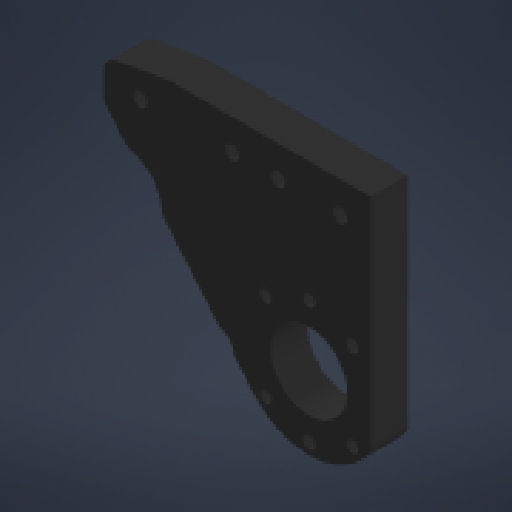
# Autodesk Inventor part: OUTSIDE_INTAKE_SPACERS
Saved by Autodesk Inventor 2026.2 (Build 302298010, 298A)
## iProperties
Created: 2026-04-02
Part Number: OUTSIDE_INTAKE_SPACERS
Material: 3D Print Material - chopped carbon Nylon12 (preferred)
Document SubType Name: Modeling
Designer: 4aida
Density: 1.05184 g/cm^3
Appearance: Black
Author: 4aida
Autodesk Inventor part; units mm, degrees
ref_plane "YZ Plane" through (0, 0, 0) normal (1, 0, 0) x (0, 1, 0)
ref_plane "XZ Plane" through (0, 0, 0) normal (0, 1, 0) x (-1, 0, 0)
ref_plane "XY Plane" through (0, 0, 0) normal (0, 0, 1) x (1, 0, 0)
sketch "Sketch1" plane through (0, 0, 0) normal (0, 0, 1) x (1, 0, 0)
  line L0 (-110, -20.8494) -> (-110, 0)
  line L1 (-110, 0) -> (0, 0)
  line L2 (0, 0) -> (0, -105)
  line L3 (0, -105) -> (-39.3892, -105)
  line L4 (-110, -20.8494) -> (-119.38, 0) construction
  line L5 (-119.38, 0) -> (-110, 0) construction
  line L6 (-50.8, -25.4) -> (0, -25.4) construction
  line L7 (0, -25.4) -> (0, 0) construction
  line L8 (0, 0) -> (-50.8, 0) construction
  line L9 (-50.8, 0) -> (-50.8, -25.4) construction
  line L10 (-50.8, -25.4) -> (0, 0) construction
  line L11 (0, -25.4) -> (-50.8, 0) construction
  circle A0 centre (-12.7, -12.7) radius 3
  circle A1 centre (-38.1, -12.7) radius 3
  circle A2 centre (-25.4, -75) radius 15.875
  circle A3 centre (-25.4, -75) radius 30
  line L12 (-50.8, -90.9637) -> (-50.8, -59.0363)
  line L13 (-110, -4.7091) -> (-83.2932, 0)
  arc A4 (-56.3982, -84.7295) -> (-61.7755, -78.3211) centre (-62.3821, -84.2903) ccw
  line L14 (-39.3892, -105) -> (-56.3982, -84.7295)
  arc A5 (-85.9963, -49.4559) -> (-100.0831, -32.6679) centre (-102.5, -49) ccw
  line L15 (-61.7755, -78.3211) -> (-85.9963, -49.4559)
  line L16 (-100.0831, -32.6679) -> (-110, -20.8494)
  circle A6 centre (-95.25, -12.7) radius 3
  circle A7 centre (-57.15, -12.7) radius 3
  point P0 (0, 0)
  point P1 (-25.4, -12.7)
  point P2 (-25.4, -25.4)
  point P3 (-50.8, -75)
  point P4 (0, -90.9637)
  point P5 (-110, -10.4247)
  point P6 (-48.3813, -94.2836)
  point P7 (0, -59.0363)
  point P8 (-25.4, -105)
  dimension "d1" = 119.38
  dimension "d2" = 50.8
  dimension "d3" = 25.4
  dimension "d4" = 25.4
  dimension "d5" = 12.7
  dimension "d6" = 6
  dimension "d7" = 6
  dimension "d11" = 110
  dimension "d12" = 60
  dimension "d13" = 25.4
  dimension "d14" = 25.4
  dimension "d17" = 20.8494
  dimension "d18" = 31.75
  dimension "d21" = 170
  dimension "d22" = 26.7068
  dimension "d24" = 86.6409
  dimension "d25" = 12
  dimension "d26" = 47.6179
  dimension "d28" = 81.3659
  dimension "d29" = 33.02
  dimension "d30" = 49
  dimension "d31" = 50
  dimension "d41" = 19.05
  dimension "d42" = 38.1
  constraints: 34 end point, 8 centre point, 6 point on circle, 5 midpoint, 4 horizontal alignment, 4 perpendicular, 4 tangent, 3 coincident, 2 collinear, 2 equal radius, 2 horizontal, 2 parallel, 2 point on line, 2 vertical, 1 vertical alignment
  measures "d1" distance from line of L2 L4.end
  measures "d2" distance of L6.start L6.end
  measures "d3" distance of L11.end L6.start
  measures "d4" distance of A1.centre A0.centre
  measures "d5" distance of point (-25.4, -12.7) A0.centre
  measures "d6" diameter of A0
  measures "d7" diameter of A1
  measures "d11" distance between parallel lines of L2 L0
  measures "d12" diameter of A3
  measures "d13" distance from line of A2.centre L2
  measures "d14" distance of point (-50.8, -75) A2.centre
  measures "d17" distance of L0.start L1.start
  measures "d18" diameter of A2
  measures "d21" angle of L13 L1
  measures "d22" horizontal distance of point (-110, -10.425) L13.end
  measures "d24" distance from line of L13 A4.centre
  measures "d25" diameter of A4
  measures "d26" distance from line of A4.centre L0
  measures "d28" distance of A5.centre A3.centre
  measures "d29" diameter of A5
  measures "d30" distance from line of L1 A5.centre
  measures "d31" angle of L1 L15
  measures "d41" distance of A1.centre A7.centre
  measures "d42" distance of A7.centre A6.centre
extrude "Extrusion1" add sketch "Sketch1" along normal blind 15.4305 contours L0 L13 L1 L2 A3 L14 A4 L15 A5 L16 | L2 A3 L12 | L12 A3
fillet "Fillet1" radius 6 8 edges at (0, -90.9637, 7.7153) (-110, -20.8494, 7.7153) (-110, -4.7091, 7.7153) (-83.2932, 0, 7.7153) (-56.3982, -84.7295, 7.7153) (-61.7755, -78.3211, 7.7153) (-85.9963, -49.4559, 7.7153) (-100.0831, -32.6679, 7.7153)
sketch "Sketch2" plane through (0, 0, 0) normal (0, 0, -1) x (-1, 0, 0)
  circle A0 centre (25.4, -75) radius 15.875 projected
  circle A1 centre (25.4, -75) radius 25.4
  line L0 (7.4395, -92.9605) -> (7.4395, -57.0395)
  line L1 (43.3605, -57.0395) -> (43.3605, -92.9605)
  line L2 (7.4395, -92.9605) -> (25.4, -75)
  line L3 (25.4, -75) -> (43.3605, -57.0395)
  point P0 (0, 0)
  point P1 (25.4, -100.4)
  point P2 (25.4, -49.6)
  dimension "d32" = 50.8
  dimension "d33" = 45
  constraints: 8 end point, 6 point on circle, 5 coincident, 2 vertical alignment, 1 centre point, 1 collinear, 1 parallel, 1 vertical
  measures "d32" diameter of A1
  measures "d33" angle of L0 L2
hole "Hole1" at (-7.4395, -92.9605, 0) at (-7.4395, -57.0395, 0) at (-43.3605, -57.0395, 0) at (-43.3605, -92.9605, 0) at (-25.4, -100.4, 0) at (-25.4, -49.6, 0) direction (0, 0, 1) diameter 5.105 end through all clearance for "Flat Head Machine Screw (82)" size "#10" standard "Ansi Unified Screw Threads"
equation "\"d5\" = 0.5 * d4"
equation "\"d7\" = d6"
equation "\"d14\" = d13"
body "Solid1"
